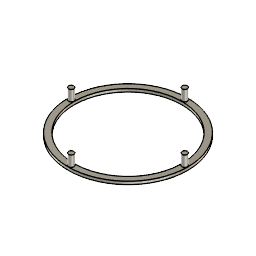
Bin leg support (Autodesk Fusion 360 design; units mm, degrees)
part number: 2026-04-06-00-43-06-802
Autodesk Fusion 360 part; units mm, degrees
sketch "Sketch1" plane through (0, 0, 0) normal (0, 0, 1) x (1, 0, 0)
  circle A0 centre (0, 0) radius 100
  circle A1 centre (0, 0) radius 90
  dimension "d1" = 200
  dimension "d2" = 180
  constraint coincident A0.centre A1.centre
  measures "d1" diameter of A0
  measures "d2" diameter of A1
extrude "Extrude1" add sketch "Sketch1" along normal blind 5
sketch "Sketch2" plane through (0, 0, 5) normal (0, 0, 1) x (-1, 0, 0)
  circle A0 centre (0, 0) radius 90
  circle A1 centre (0, 0) radius 100
  line L0 (0, 0) -> (-95, 0) construction
  line L1 (-95, 0) -> (95, 0) construction
  line L2 (95, 0) -> (95, -95) construction
  line L3 (95, -95) -> (-95, -95) construction
  line L4 (-95, -95) -> (-95, 0) construction
  line L5 (-95, 0) -> (95, 0) construction
  line L6 (95, 0) -> (95, 95) construction
  line L7 (95, 95) -> (-95, 95) construction
  line L8 (-95, 95) -> (-95, 0) construction
  circle A2 centre (95, 0) radius 4.5
  circle A3 centre (0, -95) radius 4.5
  circle A4 centre (-95, 0) radius 4.5
  circle A5 centre (0, 95) radius 4.5
  dimension "d5" = 95
  dimension "d6" = 190
  dimension "d7" = 95
  dimension "d8" = 190
  dimension "d9" = 95
  dimension "d10" = 9
  dimension "d11" = 9
  dimension "d12" = 9
  dimension "d13" = 9
  constraint coincident A0.centre A1.centre
  constraint horizontal L0
  constraint horizontal L1
  constraint vertical L2
  constraint horizontal L3
  constraint vertical L4
  constraint horizontal L5
  constraint vertical L6
  constraint horizontal L7
  constraint vertical L8
  constraint coincident L1.end L2.start
  constraint midpoint L3 A3.centre
  constraint coincident L0.end L1.start
  constraint midpoint L7 A5.centre
  measures "d5" distance of A0.centre L0.end
  measures "d6" distance of L0.end L1.end
  measures "d7" distance of L0.end L3.end
  measures "d8" distance of L0.end L1.end
  measures "d9" distance of L0.end L7.end
  measures "d10" diameter of A2
  measures "d11" diameter of A3
  measures "d12" diameter of A4
  measures "d13" diameter of A5
extrude "Extrude2" add sketch "Sketch2" along normal blind 18 contours A2 | A3 | A4 | A5
